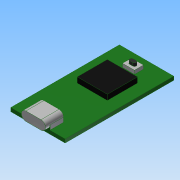
# Autodesk Inventor part: Teensy
Saved by Autodesk Inventor 2015 (Build 190159000, 159)
## iProperties
Created: 2015-08-07
Part Number: Teensy
Material: Generisch
Document SubType Name: Modeling
Designer: Johann
Density: 1 g/cm^3
Appearance: Glatt - waldgrün
Author: Johann
Autodesk Inventor part; units mm, degrees
ref_plane "YZ Plane" through (0, 0, 0) normal (1, 0, 0) x (0, 1, 0)
ref_plane "XZ Plane" through (0, 0, 0) normal (0, 1, 0) x (-1, 0, 0)
ref_plane "XY Plane" through (0, 0, 0) normal (0, 0, 1) x (1, 0, 0)
sketch "Skizze1" plane through (0, 0, 0) normal (0, 0, 1) x (1, 0, 0)
  line L0 (-9, -18) -> (9, -18)
  line L1 (9, -18) -> (9, 18)
  line L2 (9, 18) -> (-9, 18)
  line L3 (-9, 18) -> (-9, -18)
  line L4 (-9, -18) -> (9, 18) construction
  line L5 (9, -18) -> (-9, 18) construction
  point P0 (0, 0)
  dimension "d0" = 18
  dimension "d1" = 36
  constraints: 12 end point, 2 midpoint, 2 parallel, 1 horizontal, 1 perpendicular
  measures "d0" distance of L2.end L1.end
  measures "d1" distance of L1.end L0.end
extrude "Extrusion1" add sketch "Skizze1" along normal blind 1.2
sketch "Skizze5" plane through (0, 0, 1.2) normal (0, 0, 1) x (1, 0, 0)
  line L0 (4, -13.5) -> (-4, -13.5)
  line L1 (-4, -13.5) -> (-4, -19.5)
  line L2 (-4, -19.5) -> (4, -19.5)
  line L3 (4, -19.5) -> (4, -13.5)
  line L4 (4, -13.5) -> (-4, -19.5) construction
  line L5 (-4, -13.5) -> (4, -19.5) construction
  line L6 (-9, -18) -> (9, -18) projected
  point P0 (0, 0)
  point P1 (0, -16.5)
  point P2 (0, -16.5)
  dimension "d17" = 8
  dimension "d18" = 6
  dimension "d19" = 4.5
  constraints: 12 end point, 3 midpoint, 2 parallel, 1 horizontal, 1 perpendicular, 1 vertical alignment
  measures "d17" distance of L2.end L1.end
  measures "d18" distance of L1.end L0.end
  measures "d19" distance between parallel lines of L6 L0
extrude "Extrusion5" add sketch "Skizze5" along normal blind 3
fillet "Rundung1" radius 1.5 4 edges at (4, -16.5, 4.2) (-4, -16.5, 4.2) (-4, -18.75, 1.2) (4, -18.75, 1.2)
sketch "Skizze3" plane through (0, 0, 1.2) normal (0, 0, 1) x (1, 0, 0)
  line L0 (2, 12) -> (-2, 12)
  line L1 (-2, 12) -> (-2, 15)
  line L2 (-2, 15) -> (2, 15)
  line L3 (2, 15) -> (2, 12)
  line L4 (2, 12) -> (-2, 15) construction
  line L5 (-2, 12) -> (2, 15) construction
  line L6 (9, 18) -> (-9, 18) projected
  point P0 (0, 0)
  point P1 (0, 13.5)
  point P2 (0, 13.5)
  dimension "d8" = 4
  dimension "d9" = 3
  dimension "d10" = 3
  constraints: 12 end point, 3 midpoint, 2 parallel, 1 horizontal, 1 perpendicular, 1 vertical alignment
  measures "d8" distance of L1.end L2.end
  measures "d9" distance of L0.end L1.end
  measures "d10" distance between parallel lines of L6 L2
extrude "Extrusion3" add sketch "Skizze3" along normal blind 1.2
sketch "Skizze4" plane through (0, 0, 2.4) normal (0, 0, 1) x (1, 0, 0)
  line L0 (-0.5, 13.5) -> (0.5, 13.5) construction
  line L1 (-0.5, 12.9) -> (0.5, 12.9)
  line L2 (0.5, 14.1) -> (-0.5, 14.1)
  arc A0 (-0.5, 14.1) -> (-0.5, 12.9) centre (-0.5, 13.5) ccw
  arc A1 (0.5, 12.9) -> (0.5, 14.1) centre (0.5, 13.5) ccw
  line L3 (-2, 12) -> (2, 12) construction
  line L4 (2, 12) -> (2, 15) construction
  line L5 (2, 15) -> (-2, 15) construction
  line L6 (-2, 15) -> (-2, 12) construction
  line L7 (2, 15) -> (-2, 12) construction
  line L8 (-2, 15) -> (2, 12) construction
  point P0 (0, 0)
  point P1 (0, 13.5)
  point P2 (0, 13.5)
  dimension "d13" = 2.2
  dimension "d14" = 1.2
  constraints: 12 end point, 4 point on circle, 4 tangent, 2 centre point, 2 midpoint, 1 coincident, 1 horizontal, 1 parallel
  measures "d14" distance between parallel lines of L1 L2
extrude "Extrusion4" add sketch "Skizze4" along normal blind 1
sketch "Skizze2" plane through (0, 0, 1.2) normal (0, 0, 1) x (1, 0, 0)
  line L0 (5, 0) -> (-5, 0)
  line L1 (-5, 0) -> (-5, 10)
  line L2 (-5, 10) -> (5, 10)
  line L3 (5, 10) -> (5, 0)
  line L4 (5, 0) -> (-5, 10) construction
  line L5 (-5, 0) -> (5, 10) construction
  line L6 (9, 18) -> (-9, 18) projected
  point P0 (0, 0)
  point P1 (0, 5)
  dimension "d4" = 10
  dimension "d5" = 8
  constraints: 12 end point, 2 midpoint, 2 parallel, 2 perpendicular, 1 horizontal, 1 vertical alignment
  measures "d4" distance of L1.end L2.end
  measures "d5" distance between parallel lines of L6 L2
extrude "Extrusion2" add sketch "Skizze2" along normal blind 1.8
